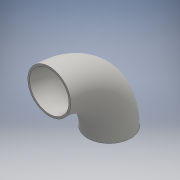
# Autodesk Inventor part: joelho 90 8 inch ANSI B16.9
Saved by Autodesk Inventor 2016 (Build 200138000, 138)
## iProperties
Created: 2018-09-12
Part Number: joelho 90 8 inch ANSI B16.9
Material: Generic
Document SubType Name: Modeling
Designer: User
Density: 1 g/cm^3
Appearance: Default
Author: User
Autodesk Inventor part; units mm, degrees
ref_plane "YZ Plane" through (0, 0, 0) normal (1, 0, 0) x (0, 1, 0)
ref_plane "XZ Plane" through (0, 0, 0) normal (0, 1, 0) x (-1, 0, 0)
ref_plane "XY Plane" through (0, 0, 0) normal (0, 0, 1) x (1, 0, 0)
sketch "Sketch4" plane through (0, 0, 0) normal (1, 0, 0) x (0, 1, 0)
  arc A0 (305, 0) -> (0, 305) centre (0, 0) ccw
  dimension "d23" = 305
  constraints: 2 point on circle, 1 centre point, 1 coincident
  measures "d23" distance of point (0, 0) A0.end
sketch "Sketch3" plane through (0, 0, 0) normal (0, 1, 0) x (-1, 0, 0)
  circle A0 centre (0, 305) radius 109.5
  circle A1 centre (0, 305) radius 99.93
  point P0 (0, 0)
  dimension "d27" = 219
  dimension "d28" = 9.57
  constraints: 2 centre point
  measures "d27" diameter of A0
  measures "d28" radial gap between concentric circles of A0 A1
sweep "Sweep6" add profiles "Sketch3" path "Sketch4"
body "Solid6"
